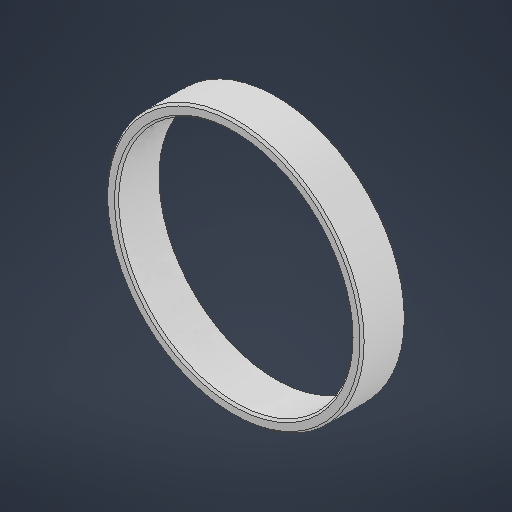
# Autodesk Inventor part: my_attempt_v2
Saved by Autodesk Inventor 2027 (Build 310192000, 192)
## iProperties
Created: 2026-05-02
Part Number: my_attempt_v2
Material: 常规
Document SubType Name: Modeling
Designer: 奎邦
Mass: 5.08846 g
Surface Area: 46.7056 cm^2
Volume: 5.08846 cm^3
Density: 1 g/cm^3
Appearance: 默认
Author: 奎邦
Autodesk Inventor part; units mm, degrees
ref_plane "YZ Plane" through (0, 0, 0) normal (1, 0, 0) x (0, 1, 0)
ref_plane "XZ Plane" through (0, 0, 0) normal (0, 1, 0) x (-1, 0, 0)
ref_plane "XY Plane" through (0, 0, 0) normal (0, 0, 1) x (1, 0, 0)
sketch "草图1" plane through (0, 0, 0) normal (0, 0, 1) x (1, 0, 0)
  circle A0 centre (0, 0) radius 30.65
  circle A1 centre (0, 0) radius 28
  constraints: 2 centre point
extrude "拉伸1" add sketch "草图1" along normal blind 10.61
chamfer "倒角1" distance 0.5 angle 45 4 edges at (-28, 0, 10.61) (-28, 0, 0) (-30.65, 0, 10.61) (-30.65, 0, 0)
